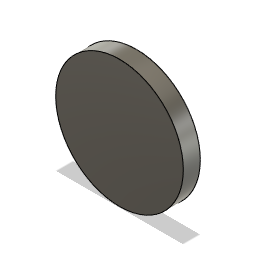
ball (Autodesk Fusion 360 design; units mm, degrees)
Autodesk Fusion 360 part; units mm, degrees
sketch "Sketch1" plane through (0, 0, 0) normal (0, 0, 1) x (1, 0, 0)
  circle A0 centre (2, 2) radius 0.75
  line L0 (2, 2) -> (2.6495, 2.375) construction
  line L1 (0, 0) -> (10, 0) construction
  dimension "jointrad" = 1.5
  dimension "ypos" = 2
  dimension "xpos" = 2
  dimension "d9" = 10
  dimension "jointangle" = 30
  constraint coincident A0.centre L0.start
  constraint coincident A0 L0.end
  constraint coincident L1.start origin
  constraint horizontal L1
  measures "jointrad" diameter of A0
  measures "ypos" vertical distance of L1.start A0.centre
  measures "xpos" horizontal distance of L1.start A0.centre
  measures "d9" distance of L1.start L1.end
  measures "jointangle" angle of L0 L1
extrude "Extrude1" add sketch "Sketch1" along normal blind 0.2
equation "jointdepth = 0.2 mm"
